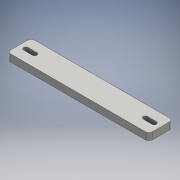
# Autodesk Inventor part: Support moteur
Saved by Autodesk Inventor 2016 (Build 200138000, 138)
## iProperties
Created: 2016-03-18
Part Number: Support moteur
Material: Generic
Document SubType Name: Modeling
Designer: Thetheos
Density: 1 g/cm^3
Appearance: Default
Author: Thetheos
Autodesk Inventor part; units mm, degrees
ref_plane "YZ Plane" through (0, 0, 0) normal (1, 0, 0) x (0, 1, 0)
ref_plane "XZ Plane" through (0, 0, 0) normal (0, 1, 0) x (-1, 0, 0)
ref_plane "XY Plane" through (0, 0, 0) normal (0, 0, 1) x (1, 0, 0)
sketch "Sketch1" plane through (0, 0, 0) normal (0, 0, 1) x (1, 0, 0)
  line L0 (0, 0) -> (160, 0)
  line L1 (160, 0) -> (160, 27)
  line L2 (160, 27) -> (0, 27)
  line L3 (0, 27) -> (0, 0)
  line L4 (152.5, 11) -> (142.5, 11)
  arc A0 (142.5, 16) -> (142.5, 11) centre (142.5, 13.5) ccw
  line L5 (142.5, 16) -> (152.5, 16)
  arc A1 (152.5, 11) -> (152.5, 16) centre (152.5, 13.5) ccw
  line L6 (7.5, 16) -> (17.5, 16)
  arc A2 (17.5, 11) -> (17.5, 16) centre (17.5, 13.5) ccw
  line L7 (17.5, 11) -> (7.5, 11)
  arc A3 (7.5, 16) -> (7.5, 11) centre (7.5, 13.5) ccw
  dimension "d0" = 160
  dimension "d1" = 27
  dimension "d2" = 10
  dimension "d3" = 10
  constraints: 16 end point, 8 point on circle, 7 tangent, 4 centre point, 3 horizontal, 2 parallel, 1 perpendicular
  measures "d0" distance of L2.end L1.end
  measures "d1" distance of L1.end L0.end
  measures "d2" distance of L4.start L4.end
  measures "d3" distance of L6.start L6.end
extrude "Extrusion1" add sketch "Sketch1" along normal blind 8
fillet "Fillet1" radius 4 4 edges at (0, 27, 4) (0, 0, 4) (160, 0, 4) (160, 27, 4)
body "Solid1"
